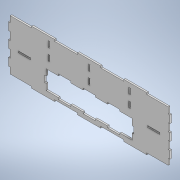
# Autodesk Inventor part: back
Saved by Autodesk Inventor 2020 (Build 240168000, 168)
## iProperties
Created: 2020-02-22
Part Number: back
Material: Generic
Document SubType Name: Modeling
Designer: udvarhelyi
Density: 1 g/cm^3
Appearance: Default
Author: udvarhelyi
Autodesk Inventor part; units mm, degrees
ref_plane "YZ Plane" through (0, 0, 0) normal (1, 0, 0) x (0, 1, 0)
ref_plane "XZ Plane" through (0, 0, 0) normal (0, 1, 0) x (-1, 0, 0)
ref_plane "XY Plane" through (0, 0, 0) normal (0, 0, 1) x (1, 0, 0)
sketch "Sketch1" plane through (0, 0, 0) normal (0, 0, 1) x (1, 0, 0)
  line L0 (-150, 14.2857) -> (-147, 14.2857)
  line L1 (-147, 28.5714) -> (-150, 28.5714)
  line L2 (-150, 42.8571) -> (-147, 42.8571)
  line L3 (-147, 57.1429) -> (-150, 57.1429)
  line L4 (-150, 71.4286) -> (-147, 71.4286)
  line L5 (-147, 85.7143) -> (-150, 85.7143)
  line L6 (147, 14.2857) -> (150, 14.2857)
  line L7 (147, 28.5714) -> (150, 28.5714)
  line L8 (150, 42.8571) -> (147, 42.8571)
  line L9 (147, 57.1429) -> (150, 57.1429)
  line L10 (150, 71.4286) -> (147, 71.4286)
  line L11 (150, 85.7143) -> (147, 85.7143)
  line L12 (-107.1429, 0) -> (-107.1429, 3)
  line L13 (-64.2857, 3) -> (-64.2857, 0)
  line L14 (-21.4286, 0) -> (-21.4286, 3)
  line L15 (21.4286, 0) -> (21.4286, 3)
  line L16 (64.2857, 0) -> (64.2857, 3)
  line L17 (107.1429, 0) -> (107.1429, 3)
  line L18 (-107.1429, 97) -> (-107.1429, 100)
  line L19 (-64.2857, 97) -> (-64.2857, 100)
  line L20 (-21.4286, 97) -> (-21.4286, 100)
  line L21 (21.4286, 97) -> (21.4286, 100)
  line L22 (64.2857, 97) -> (64.2857, 100)
  line L23 (107.1429, 97) -> (107.1429, 100)
  line L24 (-107.1429, 3) -> (-147, 3)
  line L25 (-147, 3) -> (-147, 14.2857)
  line L26 (-147, 28.5714) -> (-147, 42.8571)
  line L27 (-147, 57.1429) -> (-147, 71.4286)
  line L28 (-147, 85.7143) -> (-147, 97)
  line L29 (-147, 97) -> (-107.1429, 97)
  line L30 (-64.2857, 97) -> (-21.4286, 97)
  line L31 (21.4286, 97) -> (64.2857, 97)
  line L32 (107.1429, 97) -> (147, 97)
  line L33 (-21.4286, 3) -> (-64.2857, 3)
  line L34 (147, 3) -> (107.1429, 3)
  line L35 (64.2857, 3) -> (21.4286, 3)
  line L36 (-150, 71.4286) -> (-150, 85.7143)
  line L37 (-150, 14.2857) -> (-150, 28.5714)
  line L38 (-150, 42.8571) -> (-150, 57.1429)
  line L39 (-64.2857, 0) -> (-107.1429, 0)
  line L40 (107.1429, 0) -> (64.2857, 0)
  line L41 (21.4286, 0) -> (-21.4286, 0)
  line L42 (-107.1429, 100) -> (-64.2857, 100)
  line L43 (-21.4286, 100) -> (21.4286, 100)
  line L44 (64.2857, 100) -> (107.1429, 100)
  line L45 (150, 28.5714) -> (150, 14.2857)
  line L46 (150, 85.7143) -> (150, 71.4286)
  line L47 (150, 57.1429) -> (150, 42.8571)
  line L48 (147, 97) -> (147, 85.7143)
  line L49 (147, 71.4286) -> (147, 57.1429)
  line L50 (147, 42.8571) -> (147, 28.5714)
  line L51 (147, 14.2857) -> (147, 3)
  point P0 (0, 0)
  dimension "d1" = 300
  dimension "d5" = 42.8571
  dimension "d6" = 150
  dimension "d7" = 85.7143
  dimension "d8" = 128.5714
  dimension "d9" = 171.4286
  dimension "d10" = 214.2857
  dimension "d11" = 257.1429
  dimension "d12" = 100
  dimension "d13" = 14.2857
  dimension "d14" = 0
  dimension "d15" = 3
  dimension "d16" = 28.5714
  dimension "d17" = 42.8571
  dimension "d18" = 57.1429
  dimension "d19" = 71.4286
  dimension "d20" = 85.7143
  dimension "d21" = 94
  dimension "d22" = 3
  dimension "d23" = 3
  constraints: 104 end point, 79 perpendicular, 53 parallel, 21 collinear, 18 point on line, 3 horizontal
  measures "d1" distance of L5.end L11.start
  measures "d5" distance from line of L17.start L45
  measures "d6" distance from line of L46 point (0, 0)
  measures "d7" distance from line of L45 L16.start
  measures "d8" distance from line of L45 L15.end
  measures "d9" distance from line of L45 L14.start
  measures "d10" distance from line of L45 L13.end
  measures "d11" distance from line of L45 L12.start
  measures "d12" distance from line of L43 point (0, 0)
  measures "d13" distance from line of L0.start L39
  measures "d14" distance from line of point (0, 0) L39
  measures "d15" distance of L12.start L12.end
  measures "d16" distance from line of L39 L1.end
  measures "d17" distance from line of L39 L2.end
  measures "d18" distance from line of L39 L3.end
  measures "d19" distance from line of L39 L4.end
  measures "d20" distance from line of L39 L5.end
  measures "d21" distance between parallel lines of L24 L29
  measures "d22" distance of L11.start L11.end
  measures "d23" distance of L5.start L5.end
extrude "Extrusion1" add sketch "Sketch1" along normal blind 3
sketch "Sketch2" plane through (0, 0, 3) normal (0, 0, 1) x (1, 0, 0)
  line L0 (-80, 10) -> (80, 10)
  line L1 (80, 10) -> (80, 45)
  line L2 (80, 45) -> (-80, 45)
  line L3 (-80, 45) -> (-80, 10)
  line L4 (-21.4286, 0) -> (21.4286, 0) projected
  point P0 (0, 0)
  dimension "d26" = 80
  dimension "d27" = 80
  dimension "d28" = 35
  dimension "d29" = 10
  constraints: 8 end point, 2 parallel, 1 horizontal, 1 perpendicular
  measures "d26" distance from line of L1 point (0, 0)
  measures "d27" distance from line of point (0, 0) L3
  measures "d28" distance of L0.end L1.end
  measures "d29" distance between parallel lines of L4 L0
extrude "Extrusion2" cut sketch "Sketch2" against normal through all
sketch "Sketch4" plane through (0, 0, 3) normal (0, 0, 1) x (1, 0, 0)
  line L0 (-80, 10) -> (-80, 45) projected
  line L1 (-80, 33.3333) -> (-83, 33.3333)
  line L2 (-83, 33.3333) -> (-83, 21.6667)
  line L3 (-83, 21.6667) -> (-80, 21.6667)
  line L4 (-80, 21.6667) -> (-80, 33.3333)
  line L5 (80, 45) -> (-80, 45) projected
  line L6 (-57.1429, 45) -> (-34.2857, 45)
  line L7 (-34.2857, 45) -> (-34.2857, 48)
  line L8 (-34.2857, 48) -> (-57.1429, 48)
  line L9 (-57.1429, 48) -> (-57.1429, 45)
  line L10 (-11.4286, 45) -> (11.4286, 45)
  line L11 (11.4286, 45) -> (11.4286, 48)
  line L12 (11.4286, 48) -> (-11.4286, 48)
  line L13 (-11.4286, 48) -> (-11.4286, 45)
  line L14 (34.2857, 45) -> (57.1429, 45)
  line L15 (57.1429, 45) -> (57.1429, 48)
  line L16 (57.1429, 48) -> (34.2857, 48)
  line L17 (34.2857, 48) -> (34.2857, 45)
  line L18 (80, 33.3333) -> (83, 33.3333)
  line L19 (83, 33.3333) -> (83, 21.6667)
  line L20 (83, 21.6667) -> (80, 21.6667)
  line L21 (80, 21.6667) -> (80, 33.3333)
  line L22 (80, 45) -> (80, 10) projected
  line L23 (80, 10) -> (-80, 10) projected
  line L24 (-57.1429, 10) -> (-34.2857, 10)
  line L25 (-34.2857, 10) -> (-34.2857, 7)
  line L26 (-34.2857, 7) -> (-57.1429, 7)
  line L27 (-57.1429, 7) -> (-57.1429, 10)
  line L28 (-11.4286, 10) -> (11.4286, 10)
  line L29 (11.4286, 10) -> (11.4286, 7)
  line L30 (11.4286, 7) -> (-11.4286, 7)
  line L31 (-11.4286, 7) -> (-11.4286, 10)
  line L32 (34.2857, 10) -> (57.1429, 10)
  line L33 (57.1429, 10) -> (57.1429, 7)
  line L34 (57.1429, 7) -> (34.2857, 7)
  line L35 (34.2857, 7) -> (34.2857, 10)
  point P0 (0, 0)
  dimension "d42" = 3
  dimension "d43" = 3
  dimension "d44" = 3
  dimension "d45" = 11.6667
  dimension "d46" = 11.6667
  dimension "d47" = 22.8571
  dimension "d48" = 45.7143
  dimension "d49" = 68.5714
  dimension "d50" = 91.4286
  dimension "d51" = 114.2857
  dimension "d52" = 137.1429
  dimension "d53" = 3
  constraints: 64 end point, 16 parallel, 13 point on line, 8 horizontal, 8 perpendicular, 7 collinear
  measures "d42" distance of L1.start L1.end
  measures "d43" distance of L8.end L6.start
  measures "d44" distance of L18.start L18.end
  measures "d45" distance between parallel lines of L1 L5
  measures "d46" distance between parallel lines of L23 L3
  measures "d47" distance between parallel lines of L0 L9
  measures "d48" distance between parallel lines of L0 L7
  measures "d49" distance between parallel lines of L0 L13
  measures "d50" distance between parallel lines of L0 L11
  measures "d51" distance between parallel lines of L0 L17
  measures "d52" distance between parallel lines of L0 L15
  measures "d53" distance of L32.end L33.end
extrude "Extrusion3" cut sketch "Sketch4" against normal through all contours L13 L12 L11 L5
pattern_linear "Rectangular Pattern1" count 2 spacing 120 along (1, 0, 0) count 2 spacing 120 along (-1, 0, 0) of "Extrusion3"
extrude "Extrusion4" cut sketch "Sketch4" against normal through all contours L3 L2 L1 L0 | L23 L25 L26 L27 | L23 L29 L30 L31 | L9 L8 L7 L5 | L23 L33 L34 L35 | L17 L16 L15 L5 | L21 L18 L19 L20
sketch "Sketch5" plane through (0, 0, 3) normal (0, 0, 1) x (1, 0, 0)
  line L0 (-76.5, 92) -> (-73.5, 92)
  line L1 (-73.5, 92) -> (-73.5, 81)
  line L2 (-73.5, 81) -> (-76.5, 81)
  line L3 (-76.5, 81) -> (-76.5, 92)
  line L4 (-76.5, 70) -> (-73.5, 70)
  line L5 (-73.5, 70) -> (-73.5, 59)
  line L6 (-73.5, 59) -> (-76.5, 59)
  line L7 (-76.5, 59) -> (-76.5, 70)
  line L8 (-73.5, 92) -> (-73.5, 97) construction
  line L9 (-73.5, 81) -> (-73.5, 70) construction
  line L10 (-73.5, 59) -> (-73.5, 48) construction
  line L11 (-34.2857, 48) -> (-57.1429, 48) projected
  line L12 (-73.5, 48) -> (-57.1429, 48) construction
  line L13 (-57.1429, 48) -> (-34.2857, 48) projected
  line L14 (-73.5, 97) -> (-64.2606, 97) construction
  line L15 (-21.4286, 97) -> (-64.2857, 97) projected
  point P0 (0, 0)
  dimension "d64" = 11
  dimension "d65" = 73.5
  dimension "d66" = 3
  dimension "d72" = 11
  constraints: 26 end point, 4 collinear, 4 horizontal, 4 parallel, 3 point on line, 2 perpendicular, 2 vertical
  measures "d64" distance of L0.end L1.end
  measures "d65" distance from line of point (0, 0) L1
  measures "d66" distance of L5.end L6.end
  measures "d72" distance of L5.end L10.end
extrude "Extrusion5" cut sketch "Sketch5" against normal through all
pattern_linear "Rectangular Pattern2" count 3 spacing 75 along (1, 0, 0) of "Extrusion5"
equation "\"d1\" = wt"
equation "\"d5\" = 0.142857 * wt - tol"
equation "\"d6\" = 0.5 * wt"
equation "\"d7\" = 0.285714 * wt + tol"
equation "\"d8\" = 0.428571 * wt - tol"
equation "\"d9\" = 0.571429 * wt + tol"
equation "\"d10\" = 0.714286 * wt - tol"
equation "\"d11\" = 0.857143 * wt + tol"
equation "\"d12\" = height_front"
equation "\"d13\" = 0.142857 * height_front - tol"
equation "\"d15\" = tt"
equation "\"d16\" = 0.285714 * height_front + tol"
equation "\"d17\" = 0.428571 * height_front - tol"
equation "\"d18\" = 0.571429 * height_front + tol"
equation "\"d19\" = 0.714286 * height_front - tol"
equation "\"d20\" = 0.857143 * height_front + tol"
equation "\"d21\" = -2 * tt + height_front"
equation "\"d22\" = tt"
equation "\"d23\" = tt"
equation "\"d24\" = tt"
equation "\"d26\" = 0.5 * shelfW"
equation "\"d27\" = 0.5 * shelfW"
equation "\"d28\" = shelfH"
equation "\"tiroir\" = 1"
equation "\"d42\" = tt"
equation "\"d43\" = tt"
equation "\"d44\" = tt"
equation "\"d45\" = 0.333333 * shelfH - tol"
equation "\"d46\" = 0.333333 * shelfH - tol"
equation "\"d47\" = 0.142857 * shelfW - tol"
equation "\"d48\" = 0.285714 * shelfW + tol"
equation "\"d49\" = 0.428571 * shelfW - tol"
equation "\"d50\" = 0.571429 * shelfW + tol"
equation "\"d51\" = 0.714286 * shelfW - tol"
equation "\"d52\" = 0.857143 * shelfW + tol"
equation "\"d53\" = tt"
equation "\"d58\" = 0.4 * wt"
equation "\"d61\" = 0.4 * wt"
equation "\"d65\" = 0.25 * wt - 0.5 * tt"
equation "\"d66\" = tt"
equation "\"d71\" = 0.25 * wt"
equation "\"wt\" = 300"
equation "\"tt\" = 3"
equation "\"tol\" = 0"
equation "\"height_front\" = 100"
equation "\"d4\" = tt"
equation "\"nHoles\" = 4"
equation "\"shelfH\" = 35"
equation "\"d33\" = tt"
equation "\"shelfW\" = 160"
body "Solid1"
